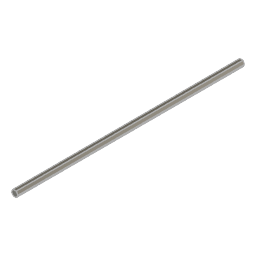
connecting rod bottom (Autodesk Fusion 360 design; units mm, degrees)
Autodesk Fusion 360 part; units mm, degrees
sketch "Sketch1" plane through (0, 0, 0) normal (0, 1, 0) x (1, 0, 0)
  line L0 (2.8868, 0) -> (1.4434, 2.5)
  line L1 (1.4434, 2.5) -> (-1.4434, 2.5)
  line L2 (-1.4434, 2.5) -> (-2.8868, 0)
  line L3 (-2.8868, 0) -> (-1.4434, -2.5)
  line L4 (-1.4434, -2.5) -> (1.4434, -2.5)
  line L5 (1.4434, -2.5) -> (2.8868, 0)
  dimension "d1" = 2.5
  constraint horizontal L1
  measures "d1" distance of origin L5
extrude "Extrude1" add sketch "Sketch1" along normal blind 200
named bodies: "rod"
